Autodesk Fusion 360 part; units mm, degrees
(part 2 of 2)
sketch "Sketch1" plane through (0, 0, 0) normal (0, 0, 1) x (1, 0, 0)
  line L0 (17, -26) -> (-17, -26)
  line L1 (-17, -26) -> (-17, 26)
  line L2 (-17, 26) -> (17, 26)
  line L3 (17, 26) -> (17, -26)
  line L4 (17, -26) -> (-17, 26) construction
  line L5 (-17, -26) -> (17, 26) construction
  line L6 (-17, 26) -> (-15.5, 26)
  line L7 (-15.5, 26) -> (-15.5, 27.5)
  line L8 (-15.5, 27.5) -> (-17, 27.5)
  line L9 (-17, 27.5) -> (-17, 26)
  line L10 (-17, 26) -> (-18.8, 26)
  line L11 (-18.8, 26) -> (-18.8, 27.5)
  line L12 (-18.8, 27.5) -> (-17, 27.5)
  line L13 (-17, 27.5) -> (-17, 26)
  line L14 (-18.8, 26) -> (-17, 26)
  line L15 (-17, 26) -> (-17, 24.7)
  line L16 (-17, 24.7) -> (-18.8, 24.7)
  line L17 (-18.8, 24.7) -> (-18.8, 26)
  dimension "d7" = 34
  dimension "d8" = 52
  dimension "d13" = 1.5
  dimension "d14" = 1.5
  dimension "d15" = 1.5
  constraint horizontal L0
  constraint perpendicular L0 L1
  constraint parallel L0 L2
  constraint parallel L1 L3
  constraint coincident L4 origin
  constraint coincident L5 origin
  constraint horizontal L6
  constraint vertical L7
  constraint horizontal L8
  constraint vertical L9
  constraint horizontal L10
  constraint vertical L11
  constraint horizontal L12
  constraint vertical L13
  constraint horizontal L14
  constraint vertical L15
  constraint horizontal L16
  constraint vertical L17
  constraint coincident L1 L15.end
  measures "d7" distance of L1.end L2.end
  measures "d8" distance of L0.end L1.end
  measures "d13" distance of L1.end L6.end
  measures "d14" distance of L1.end L8.end
  measures "d15" distance of L1.end L8.end
extrude "Extrude3" add sketch "Sketch1" along normal blind 5 contours L0 L1 L2 L3 L6 L15
extrude "Extrude4" add sketch "Sketch1" along normal blind 3 from surface at 2 contours L1 L10 L14 L15 L16 L17 | L2 L6 L7 L8 L9 L13 | L9 L10 L11 L12 L13 L14
equation "d15 = d14"

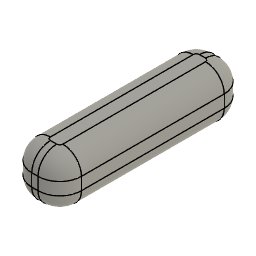
design "PTFE Magnetic Stirrer Bar"
Autodesk Fusion 360 part; units mm, degrees
sketch "Sketch1" plane through (0, 0, 0) normal (0, 1, 0) x (1, 0, 0)
  line L0 (0, 0) -> (8, 0)
  line L1 (8, 0) -> (8, -8)
  line L2 (8, -8) -> (0, -8)
  line L3 (0, -8) -> (0, 0)
  dimension "d1" = 8
  dimension "d2" = 8
  constraint horizontal L0
  constraint vertical L1
  constraint horizontal L2
  constraint vertical L3
  constraint coincident L0.start L3.end
  measures "d1" distance of L0.start L0.end
  measures "d2" distance of L0.start L2.end
extrude "Extrude1" add sketch "Sketch1" along normal blind 30
fillet "Fillet1" radius 3.5 4 edges at (8, 0, 4) (0, 0, 4) (0, 30, 4) (8, 30, 4)
fillet "Fillet2" radius 3 16 edges at (6.9749, 28.9749, 8) (4, 30, 8) (1.0251, 28.9749, 8) (0, 15, 8) (1.0251, 1.0251, 8) (4, 0, 8) (6.9749, 1.0251, 8) (8, 15, 8) (4, 30, 0) (1.0251, 28.9749, 0) (0, 15, 0) (1.0251, 1.0251, 0) (4, 0, 0) (6.9749, 1.0251, 0) (8, 15, 0) (6.9749, 28.9749, 0)

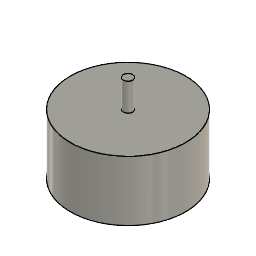
design "R300C DC Motor"
Autodesk Fusion 360 part; units mm, degrees
sketch "Sketch1" plane through (0, 0, 0) normal (0, 0, 1) x (1, 0, 0)
  circle A0 centre (0, 0) radius 12
  dimension "d1" = 24
  constraint coincident A0.centre origin
  measures "d1" diameter of A0
extrude "Extrude1" add sketch "Sketch1" along normal blind 12.5
sketch "Sketch2" plane through (0, 0, 12.5) normal (0, 0, 1) x (-1, 0, 0)
  circle A0 centre (0, 0) radius 12
  circle A1 centre (0, 0) radius 1
  dimension "d4" = 2
  constraint coincident A0.centre A1.centre
  measures "d4" diameter of A1
extrude "Extrude2" add sketch "Sketch2" along normal blind 5.75 contours A1

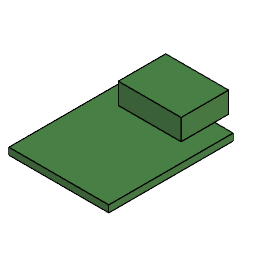
design "Type-C Lithium Battery Charger Board"
Autodesk Fusion 360 part; units mm, degrees
sketch "Sketch1" plane through (0, 0, 0) normal (0, 0, 1) x (1, 0, 0)
  line L0 (-7.15, 8.9) -> (7.15, 8.9)
  line L1 (7.15, 8.9) -> (7.15, -8.9)
  line L2 (7.15, -8.9) -> (-7.15, -8.9)
  line L3 (-7.15, -8.9) -> (-7.15, 8.9)
  line L4 (-7.15, 8.9) -> (7.15, -8.9) construction
  line L5 (7.15, 8.9) -> (-7.15, -8.9) construction
  dimension "d13" = 14.3
  dimension "d14" = 17.8
  constraint horizontal L0
  constraint perpendicular L0 L1
  constraint parallel L0 L2
  constraint parallel L1 L3
  constraint coincident L4 origin
  constraint coincident L5 origin
  measures "d13" distance of L1.end L2.end
  measures "d14" distance of L0.end L1.end
extrude "Extrude5" add sketch "Sketch1" along normal blind 1
sketch "Sketch3" plane through (0, 0, 1) normal (0, 0, 1) x (-1, 0, 0)
  line L0 (7.15, 8.9) -> (-7.15, 8.9)
  line L1 (-7.15, 8.9) -> (-7.15, -8.9)
  line L2 (-7.15, -8.9) -> (7.15, -8.9)
  line L3 (7.15, -8.9) -> (7.15, 8.9)
  line L4 (0, -8.9) -> (0, -10.9)
  line L5 (4.5, -10.9) -> (-4.5, -10.9)
  line L6 (4.5, -10.9) -> (4.5, -4.1)
  line L7 (4.5, -4.1) -> (-4.5, -4.1)
  line L8 (-4.5, -4.1) -> (-4.5, -10.9)
  dimension "d17" = 2
  dimension "d18" = 4.5
  dimension "d19" = 9
  dimension "d20" = 6.8
  constraint midpoint L2 L4.start
  constraint perpendicular L2 L4
  constraint perpendicular L5 L6
  constraint perpendicular L6 L7
  constraint perpendicular L5 L8
  measures "d17" distance of L4.start L4.end
  measures "d18" distance of L4.end L5.start
  measures "d19" distance of L5.start L5.end
  measures "d20" distance of L5.start L6.end
extrude "Extrude6" add sketch "Sketch3" along normal blind 3 contours L2 L4 L5 L6 | L2 L6 L7 L8 | L2 L4 L5 L8
